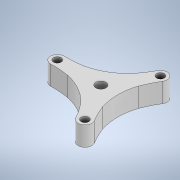
# Autodesk Inventor part: stability
Saved by Autodesk Inventor 2020 (Build 240168000, 168)
## iProperties
Created: 2019-07-11
Part Number: stability
Material: Generic
Document SubType Name: Modeling
Designer: ColinP
Density: 1 g/cm^3
Appearance: Default
Author: ColinP
Autodesk Inventor part; units mm, degrees
ref_plane "YZ Plane" through (0, 0, 0) normal (1, 0, 0) x (0, 1, 0)
ref_plane "XZ Plane" through (0, 0, 0) normal (0, 1, 0) x (-1, 0, 0)
ref_plane "XY Plane" through (0, 0, 0) normal (0, 0, 1) x (1, 0, 0)
sketch "Sketch1" plane through (0, 0, 0) normal (0, 1, 0) x (-1, 0, 0)
  line L0 (0, 0) -> (28.575, 0)
  line L1 (28.575, 0) -> (0, 0)
  line L2 (0, 0) -> (-14.2875, -24.746676)
  line L3 (0, 0) -> (28.575, 0) construction
  line L4 (0, 0) -> (-14.2875, 24.746676)
  line L5 (0, 0) -> (28.575, 0) construction
  circle A0 centre (28.575, 0) radius 2.54
  circle A1 centre (-14.2875, -24.746676) radius 2.54
  circle A2 centre (-14.2875, 24.746676) radius 2.54
  circle A3 centre (0, 0) radius 3.175
  dimension "d0" = 28.575
  dimension "d1" = 28.575
  dimension "d2" = 120
  dimension "d3" = 28.575
  dimension "d4" = 120
  dimension "d5" = 5.08
  dimension "d6" = 5.08
  dimension "d7" = 5.08
  dimension "d9" = 6.35
  constraints: 12 end point, 4 centre point, 4 coincident, 3 horizontal, 2 equal length, 1 collinear
  measures "d0" distance of L0.start L0.end
  measures "d1" distance of L0.start L2.end
  measures "d2" angle of L2 L3
  measures "d3" distance of L0.start L4.end
  measures "d4" angle of L5 L4
  measures "d5" diameter of A0
  measures "d6" diameter of A1
  measures "d7" diameter of A2
  measures "d9" diameter of A3
sketch "Sketch2" plane through (0, 0, 0) normal (0, 1, 0) x (-1, 0, 0)
  circle A0 centre (28.575, 0) radius 2.54
  circle A1 centre (-14.2875, -24.746676) radius 2.54
  circle A2 centre (-14.2875, 24.746676) radius 2.54
  circle A3 centre (28.575, 0) radius 4.445
  circle A4 centre (-14.2875, -24.746676) radius 4.445
  circle A5 centre (-14.2875, 24.746676) radius 4.445
  circle A6 centre (0, 0) radius 6.35
  circle A7 centre (0, 0) radius 9.525
  line L0 (28.575, 4.445) -> (28.575, -4.445)
  line L1 (-14.2875, 24.746676) -> (0, 0)
  line L2 (0, 0) -> (-14.2875, 24.746676)
  line L3 (-14.2875, 24.746676) -> (-10.438017, 26.969176)
  line L4 (-14.2875, 24.746676) -> (-18.136983, 22.524176)
  line L5 (0, 0) -> (-14.2875, -24.746676)
  line L6 (-10.438017, -26.969176) -> (-14.2875, -24.746676)
  line L7 (-18.136983, -22.524176) -> (-14.2875, -24.746676)
  arc A8 (4.7625, 8.248892) -> (28.575, 4.445) centre (26.99693, 71.00172) ccw
  arc A9 (28.575, -4.445) -> (4.7625, -8.248892) centre (26.881025, -70.276152) ccw
  arc A10 (4.7625, -8.248892) -> (-10.438017, -26.969176) centre (47.42042, -58.417726) ccw
  arc A11 (-18.136983, -22.524176) -> (-9.525, 0) centre (-74.301445, 11.858426) ccw
  arc A12 (-9.525, 0) -> (-18.136983, 22.524176) centre (-78.365024, -13.41211) ccw
  arc A13 (-10.438017, 26.969176) -> (4.7625, 8.248892) centre (47.42042, 58.417726) ccw
  arc A14 (-3.701951, 16.907326) -> (16.495087, 5.259811) centre (24.822359, 43.03428) ccw
  arc A15 (16.493149, -5.24768) -> (-3.701951, -16.907326) centre (24.881633, -43.096252) ccw
  line L8 (-9.525, 0) -> (-10.9982, 0)
  arc A16 (-12.791199, -11.659646) -> (-12.855666, 11.634998) centre (-49.072802, -0.112643) ccw
  dimension "d10" = 8.89
  dimension "d11" = 8.89
  dimension "d12" = 8.89
  dimension "d13" = 12.7
  dimension "d14" = 19.05
  dimension "d15" = 1.4732
  constraints: 31 point on circle, 18 end point, 14 centre point, 5 coincident, 3 perpendicular, 1 collinear, 1 horizontal, 1 line through centre, 1 point on line, 1 vertical
  measures "d10" diameter of A3
  measures "d11" diameter of A4
  measures "d12" diameter of A5
  measures "d13" diameter of A6
  measures "d14" diameter of A7
  measures "d15" distance of L8.start L8.end
sketch "Sketch2 outline for Extrusion1" plane through (0, 0, 0) normal (0, 1, 0) x (-1, 0, 0)
  arc A0 (-10.438017, 26.969176) -> (-18.136983, 22.524176) centre (-14.2875, 24.746676) ccw
  arc A1 (-3.701951, 16.907326) -> (-10.438017, 26.969176) centre (47.42042, 58.417726) cw
  arc A2 (-18.136983, 22.524176) -> (-12.855666, 11.634998) centre (-78.365024, -13.41211) cw
  arc A3 (16.495087, 5.259811) -> (-3.701951, 16.907326) centre (24.822359, 43.03428) cw
  arc A4 (-12.855666, 11.634998) -> (-12.791199, -11.659646) centre (-49.072802, -0.112643) cw
  arc A5 (28.575, 4.445) -> (16.495087, 5.259811) centre (26.99693, 71.00172) cw
  arc A6 (-12.791199, -11.659646) -> (-18.136983, -22.524176) centre (-74.301445, 11.858426) cw
  arc A7 (28.575, -4.445) -> (28.575, 4.445) centre (28.575, 0) ccw
  arc A8 (-18.136983, -22.524176) -> (-10.438017, -26.969176) centre (-14.2875, -24.746676) ccw
  arc A9 (16.493149, -5.24768) -> (28.575, -4.445) centre (26.881025, -70.276152) cw
  arc A10 (-10.438017, -26.969176) -> (-3.701951, -16.907326) centre (47.42042, -58.417726) cw
  arc A11 (-3.701951, -16.907326) -> (16.493149, -5.24768) centre (24.881633, -43.096252) cw
  circle A12 centre (-14.2875, -24.746676) radius 2.54
  circle A13 centre (-14.2875, 24.746676) radius 2.54
  circle A14 centre (28.575, 0) radius 2.54
extrude "Extrusion1" add sketch "Sketch2 outline for Extrusion1" along normal blind 12.7
hole "Hole1" at (0, 0, 0) direction (0, 1, 0) diameter 6.35 end through all
sketch "Sketch3" plane through (0, 12.7, 0) normal (0, 1, 0) x (1, 0, 0)
  circle A0 centre (0, 0) radius 3.175 projected
  constraints: 1 coincident
hole "Hole2" at (0, 12.7, 0) direction (0, -1, 0) diameter 6.604 end through all
body "Solid1"
